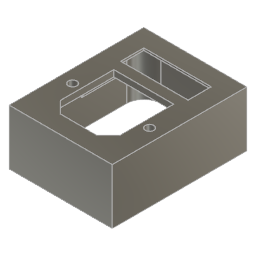
PC plug and switch housing v2 (Autodesk Fusion 360 design; units mm, degrees)
Autodesk Fusion 360 part; units mm, degrees
note: some values were not read from the file. Set by a fixed rule: which sketch regions a step uses.
sketch "Sketch1" plane through (0, 0, 0) normal (0, 0, 1) x (1, 0, 0)
  line L0 (0, 0) -> (28, 0) construction
  line L1 (28, 0) -> (28, 30.5) construction
  line L2 (28, 30.5) -> (0, 30.5)
  line L3 (0, 30.5) -> (0, 0) construction
  line L4 (5.5, 0) -> (22.5, 0)
  line L5 (28, 30.5) -> (28, 5.5)
  line L6 (28, 5.5) -> (0, 5.5) construction
  line L7 (22.5, 0) -> (28, 5.5)
  line L8 (5.5, 0) -> (0, 5.5)
  line L9 (0, 30.5) -> (0, 5.5)
  line L10 (14, 30.5) -> (14, 35.5) construction
  line L11 (-1.75, 46.3) -> (29.75, 46.3)
  line L12 (29.75, 46.3) -> (29.75, 35.5)
  line L13 (29.75, 35.5) -> (-1.75, 35.5)
  line L14 (-1.75, 35.5) -> (-1.75, 46.3)
  line L15 (-1.75, 35.5) -> (-1.75, 0) construction
  line L16 (29.75, 35.5) -> (29.75, 0) construction
  line L17 (0, 0) -> (-1.75, 0) construction
  line L18 (28, 0) -> (29.75, 0) construction
  line L19 (-10.15, 35.5) -> (-10.15, 54.7)
  line L20 (-10.15, 54.7) -> (38.15, 54.7)
  line L21 (38.15, 54.7) -> (38.15, 35.5)
  line L22 (38.15, 35.5) -> (38.15, -8.4)
  line L23 (28, -8.4) -> (38.15, -8.4)
  line L24 (0, -8.4) -> (28, -8.4)
  line L25 (0, -8.4) -> (-10.15, -8.4)
  line L26 (-10.15, 35.5) -> (-10.15, -8.4)
  line L27 (32, 15.25) -> (28, 15.25) construction
  circle A0 centre (32, 15.25) radius 2
  line L28 (28, 15.25) -> (0, 15.25) construction
  line L29 (0, 15.25) -> (-4, 15.25) construction
  circle A1 centre (-4, 15.25) radius 2
  line L30 (-9.15, 35.5) -> (-9.15, -7.4)
  line L31 (0, -7.4) -> (-9.15, -7.4)
  line L32 (0, -7.4) -> (28, -7.4)
  line L33 (28, -7.4) -> (37.15, -7.4)
  line L34 (37.15, 35.5) -> (37.15, -7.4)
  line L35 (37.15, 53.7) -> (37.15, 35.5)
  line L36 (-9.15, 53.7) -> (37.15, 53.7)
  line L37 (-9.15, 35.5) -> (-9.15, 53.7)
  line L38 (32, 15.25) -> (38.15, 15.25) construction
  line L39 (-4, 15.25) -> (-10.15, 15.25) construction
  line L40 (38.15, 19.25) -> (38.15, 11.25) construction
  line L41 (38.15, 11.25) -> (37.15, 11.25)
  line L42 (37.15, 11.25) -> (37.15, 19.25)
  line L43 (37.15, 19.25) -> (38.15, 19.25)
  line L44 (38.15, 19.25) -> (38.15, 11.25)
  line L45 (-10.15, 19.25) -> (-10.15, 11.25) construction
  line L46 (-10.15, 11.25) -> (-10.15, 19.25)
  line L47 (-10.15, 19.25) -> (-8.15, 19.25)
  line L48 (-8.15, 19.25) -> (-8.15, 11.25)
  line L49 (-8.15, 11.25) -> (-10.15, 11.25)
  line L50 (38.15, 11.25) -> (38.15, 19.25)
  line L51 (38.15, 19.25) -> (36.15, 19.25)
  line L52 (36.15, 19.25) -> (36.15, 11.25)
  line L53 (36.15, 11.25) -> (38.15, 11.25)
  line L54 (37.15, 33.5) -> (-9.15, 33.5)
  line L55 (-9.15, 33.5) -> (-9.15, 32.5)
  line L56 (-9.15, 32.5) -> (37.15, 32.5)
  line L57 (37.15, 32.5) -> (37.15, 33.5)
  line L58 (37.15, 33.5) -> (-9.15, 32.5) construction
  line L59 (-9.15, 33.5) -> (37.15, 32.5) construction
  point P0 (14, 33)
  dimension "d1" = 28
  dimension "d2" = 30.5
  dimension "d3" = 17
  dimension "d4" = 25
  dimension "d5" = 5
  dimension "d7" = 31.5
  dimension "d8" = 10.8
  dimension "d9" = 8.4
  dimension "d10" = 4
  dimension "d11" = 4
  dimension "d13" = 4
  dimension "d14" = 4
  dimension "d17" = 7.4
  dimension "d18" = 8
  dimension "d19" = 8
  dimension "d23" = 1
  measures "d1" distance of L0.start L0.end
  measures "d2" distance of L0.start L2.end
  measures "d3" distance of L4.start L4.end
  measures "d4" distance of L1.end L5.end
  measures "d5" distance of L10.start L10.end
  measures "d7" distance of L11.start L11.end
  measures "d8" distance of L11.start L13.end
  measures "d10" distance of L27.start L27.end
  measures "d11" diameter of A0
  measures "d13" distance of L28.end L29.end
  measures "d14" diameter of A1
  measures "d18" distance of L40.start L40.end
  measures "d19" distance of L45.start L45.end
  measures "d23" distance of L54.end L55.end
extrude "Extrude1" add sketch "Sketch1" along normal blind 1 makes body 1
extrude "Extrude2" add sketch "Sketch1" against normal blind 25 separate body contours L19 L20 L21 L22 L26 L30 L34 L35 L36 L37 L43 L47 L51 L55 L57 | L26 L30 L46 L47 L49 | L22 L23 L24 L25 L26 L30 L31 L32 L33 L34 L41 L49 L53 | L22 L34 L41 L42 L43 L44 L50 L51 L53 makes body 2
fillet "Fillet1" radius 8 4 edges at (37.15, -7.4, -12.5) (37.15, 53.7, -12.5) (-9.15, 53.7, -12.5) (-9.15, -7.4, -12.5) on bodies 2
combine "Combine1" operation add target body 1 tool bodies 2
extrude "Extrude3" add sketch "Sketch1" against normal blind 4 contours L30 L34 L54 L55 L56 L57 bodies 1
fillet "Fillet2" radius 8 4 edges at (-9.15, 33.5, -2) (-9.15, 32.5, -2) (37.15, 32.5, -2) (37.15, 33.5, -2) on bodies 1
fillet "Fillet3" radius 8 2 edges at (37.15, 33, -4) (-9.15, 33, -4) on bodies 1
fillet "Fillet4" radius 1.999 8 edges at (-6.8069, 35.8431, 0) (-9.15, 43.6, 0) (-6.8069, 51.3569, 0) (14, 53.7, 0) (34.8069, 51.3569, 0) (37.15, 43.6, 0) (34.8069, 35.8431, 0) (14, 33.5, 0) on bodies 1
fillet "Fillet5" radius 0.5 3 edges at (-6.8069, 35.8431, -6.3431) (14, 33.5, -4) (34.8069, 35.8431, -6.3431) on bodies 1
fillet "Fillet6" radius 0.5 3 edges at (34.8069, 30.1569, -6.3431) (14, 32.5, -4) (-6.8069, 30.1569, -6.3431) on bodies 1
extrude "Extrude4" add 1 faces at (16.8333, -4.9333, 0) along direction (0, 0, -1) blind 2 on bodies 1 bodies 1
equation "d17 = 8.4 mm - 1 mm"
named bodies: "PC Plug and switch housing"
